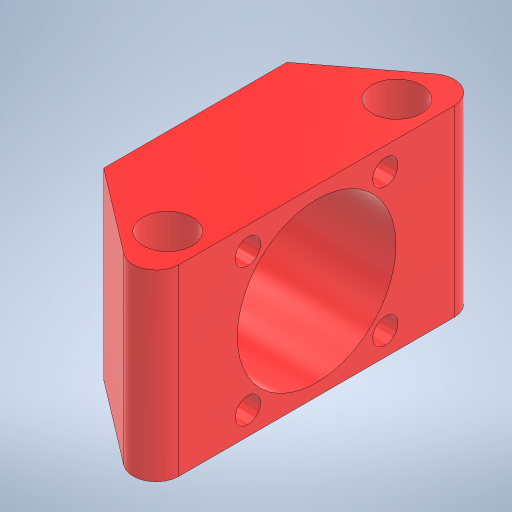
# Autodesk Inventor part: Motor Sleeve
Saved by Autodesk Inventor 2023.2 (Build 272271000, 271)
## iProperties
Created: 2022-12-29
Part Number: Motor Sleeve
Material: UHMW, Black
Document SubType Name: Modeling
Designer: Nathan Cai
Density: 0.94 g/cm^3
Appearance: Light Red
Mass: 6.50335 g
Surface Area: 59.7627 cm^2
Volume: 6.91846 cm^3
Author: Nathan Cai
Autodesk Inventor part; units mm, degrees
ref_plane "YZ Plane" through (0, 0, 0) normal (1, 0, 0) x (0, 1, 0)
ref_plane "XZ Plane" through (0, 0, 0) normal (0, 1, 0) x (-1, 0, 0)
ref_plane "XY Plane" through (0, 0, 0) normal (0, 0, 1) x (1, 0, 0)
sketch "Sketch1" plane through (0, 0, 0) normal (1, 0, 0) x (0, 1, 0)
  circle A0 centre (0, 0) radius 11
  line L0 (-12.7, 12.7) -> (12.7, 12.7)
  line L1 (12.7, 12.7) -> (12.7, -12.7)
  line L2 (12.7, -12.7) -> (-12.7, -12.7)
  line L3 (-12.7, -12.7) -> (-12.7, 12.7)
  line L4 (-12.7, 12.7) -> (12.7, -12.7) construction
  line L5 (12.7, 12.7) -> (-12.7, -12.7) construction
  line L6 (-9.525, 9.525) -> (9.525, 9.525) construction
  line L7 (9.525, 9.525) -> (9.525, -9.525) construction
  line L8 (9.525, -9.525) -> (-9.525, -9.525) construction
  line L9 (-9.525, -9.525) -> (-9.525, 9.525) construction
  line L10 (-9.525, 9.525) -> (9.525, -9.525) construction
  line L11 (9.525, 9.525) -> (-9.525, -9.525) construction
  circle A1 centre (9.525, 9.525) radius 1.7526
  circle A2 centre (-9.525, 9.525) radius 1.7526
  circle A3 centre (-9.525, -9.525) radius 1.7526
  circle A4 centre (9.525, -9.525) radius 1.7526
  dimension "d0" = 22
  dimension "d1" = 25.4
  dimension "d2" = 25.4
  dimension "d3" = 19.05
  dimension "d4" = 19.05
  dimension "d5" = 3.5052
  dimension "d8" = 360
  constraints: 24 end point, 5 centre point, 4 midpoint, 4 parallel, 2 coincident, 2 horizontal, 2 perpendicular, 9 other
  measures "d0" diameter of A0
  measures "d1" distance of L1.end L2.end
  measures "d2" distance of L0.end L1.end
  measures "d3" distance of L7.end L8.end
  measures "d4" distance of L6.end L7.end
  measures "d5" diameter of A1
extrude "Extrusion1" add sketch "Sketch1" along normal blind 16.8
sketch "Sketch2" plane through (0, 12.7, 12.7) normal (0, 1, 0) x (1, 0, 0)
  circle A0 centre (12.0375, -3.175) radius 4.7625
  circle A1 centre (12.0375, -3.175) radius 3.175
  line L0 (0, 0) -> (16.8, 0) projected
  line L1 (16.8, 25.4) -> (16.8, 0) projected
  line L2 (0, 12.7) -> (16.8, 12.7) construction
  line L3 (16.8, -12.7833) -> (16.8, 0)
  circle A2 centre (12.0375, 28.575) radius 4.7625
  circle A3 centre (12.0375, 28.575) radius 3.175
  line L4 (0, 25.4) -> (16.8, 25.4)
  line L5 (16.8, 38.1833) -> (16.8, 25.4)
  line L6 (0, 25.4) -> (16.8, 25.4) projected
  line L7 (0, 25.4) -> (16.8, 38.1833)
  line L8 (0, 0) -> (16.8, -12.7833)
  point P0 (16.8, -3.175)
  point P1 (16.8, 28.575)
  point P2 (15.5873, 25.4)
  point P3 (8.4877, 25.4)
  point P4 (9.1536, -6.9651)
  point P5 (8.4877, 0)
  point P6 (15.5873, 0)
  dimension "d12" = 9.525
  dimension "d13" = 6.35
  constraints: 12 end point, 4 symmetric about line, 3 point on line, 2 centre point, 2 coincident, 2 vertical, 1 horizontal, 1 midpoint, 1 perpendicular, 1 tangent, 9 other
  measures "d13" diameter of A1
extrude "Extrusion2" add sketch "Sketch2" against normal up to surface (25.4 mm away) contours A0 L0 | L3 L8 A0 | A0 L0 L3 | L8 L0 A0 | A2 L4 | L5 L4 A2 | A2 L7 L5 | A2 L4 L7 | A2 L4 picked at (16.2227, -3.5628)
thicken "Thicken1" operation cut thickness 0.254 both sides no extend neighbours no toward (0.9967573, 0, 0.0804666) faces at (15.2022, -4.2333, 16.1305)
thicken "Thicken2" operation cut thickness 0.254 both sides no extend neighbours no toward (0.9870503, 0, -0.1604113) faces at (15.1714, 4.2333, -16.3843)
fillet "Fillet4" radius 3.175 2 edges at (16.8, 0, 25.4833) (16.8, 0, -25.4833)
body "Solid1"
